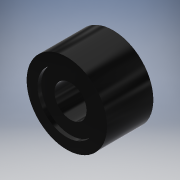
# Autodesk Inventor part: 膝_同軸_スペーサ_1_2
Saved by Autodesk Inventor 2018 (Build 220112000, 112)
## iProperties
Created: 2016-05-01
Part Number: 膝_同軸_スペーサ_1_2
Material: アセタール樹脂、黒
Document SubType Name: Modeling
Designer: hiroaki
Density: 1.425 g/cm^3
Appearance: 滑らか - 黒
Mass: 0.567513 g
Surface Area: 4.48604 cm^2
Volume: 0.398255 cm^3
Author: hiroaki
Autodesk Inventor part; units mm, degrees
ref_plane "YZ Plane" through (0, 0, 0) normal (1, 0, 0) x (0, 1, 0)
ref_plane "XZ Plane" through (0, 0, 0) normal (0, 1, 0) x (-1, 0, 0)
ref_plane "XY Plane" through (0, 0, 0) normal (0, 0, 1) x (1, 0, 0)
sketch "スケッチ1" plane through (0, 0, 0) normal (0, 0, 1) x (1, 0, 0)
  line L0 (2.6, 3.45) -> (2.6, -3.45)
  line L1 (2.6, -3.45) -> (6.5, -3.45)
  line L2 (6.5, -3.45) -> (6.5, 3.45)
  line L3 (6.5, 3.45) -> (2.6, 3.45)
  line L4 (0, -5.55) -> (0, 4.95) projected
  line L5 (6.5, -3.45) -> (4.75, -3.45)
  line L6 (4.75, -3.45) -> (4.75, -4.05)
  line L7 (4.75, -4.05) -> (6.5, -4.05)
  line L8 (6.5, -4.05) -> (6.5, -3.45)
  point P0 (0, 0)
  point P1 (2.6, 0)
  dimension "d1" = 2.6
  dimension "d2" = 6.5
  dimension "d3" = 6.9
  dimension "d8" = 0.6
  dimension "d9" = 4.75
  constraints: 16 end point, 4 perpendicular, 2 parallel, 1 horizontal, 1 horizontal alignment, 1 midpoint, 1 vertical
  measures "d1" distance from line of point (0, 0) L0
  measures "d2" distance from line of point (0, 0) L2
  measures "d3" distance of L1.end L2.end
  measures "d8" distance of L7.end L1.end
  measures "d9" distance between parallel lines of L4 L6
revolve "回転1" add sketch "スケッチ1" angle 360 about axis through (0, -10, 0) along (0, 1, 0)
